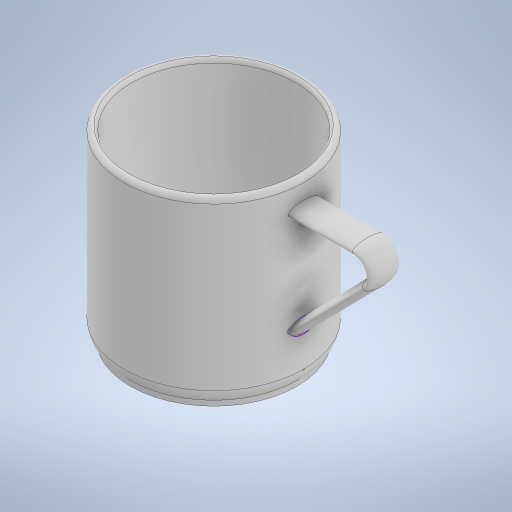
# Autodesk Inventor part: Lab No. 2
Saved by Autodesk Inventor 2024 (Build 280153000, 153)
## iProperties
Created: 2024-02-22
Part Number: Lab No. 2
Material: Generic
Document SubType Name: Modeling
Designer: Admin
Density: 1 g/cm^3
Appearance: Default
Author: Admin
Autodesk Inventor part; units mm, degrees
sketch "Sketch1" plane through (0, 0, 0) normal (0, 0, 1) x (1, 0, 0)
  line L0 (0, 0) -> (0, 70)
  line L1 (0, 70) -> (-35, 70)
  line L2 (-35, 70) -> (-35, 5)
  line L3 (0, 0) -> (-32.5, 0)
  arc A0 (-35, 5) -> (-32.5, 0) centre (-28.75, 5) ccw
  dimension "d0" = 70
  dimension "d1" = 35
  dimension "d2" = 65
  dimension "d3" = 32.5
  constraints: 8 end point, 2 perpendicular, 2 point on circle, 1 centre point, 1 horizontal, 1 tangent, 1 vertical
  measures "d0" distance of L0.start L0.end
  measures "d1" distance of L0.end L1.end
  measures "d2" distance of L1.end L2.end
  measures "d3" distance of L0.start L3.end
revolve "Revolution1" add sketch "Sketch1" angle 360 about axis through (0, 0, 0) along (0, 1, 0)
shell "Shell1" thickness 3 removed faces 1 at (-0.2748, 70, -9.3581)
sketch "Sketch2" plane through (0, 0, 0) normal (0, 0, 1) x (1, 0, 0)
  line L0 (35, 60) -> (60, 60)
  line L1 (35, 20) -> (64.0906, 49.6106)
  line L2 (35, 5) -> (35, 70) projected
  arc A0 (64.0906, 49.6106) -> (60, 60) centre (60, 54) ccw
  constraints: 4 end point, 2 point on circle, 1 centre point
ref_plane "Work Plane1" through (35, 60, 0) normal (1, 0, 0) x (0, 1, 0)
sketch "Sketch3" plane through (35, 60, 0) normal (1, 0, 0) x (0, 1, 0)
  ellipse E0 centre (0, 0) end of major axis (0, -6) minor radius 2
  point P0 (-60, 0)
  constraints: 2 other
ref_plane "Work Plane2" through (35, 5, 0) normal (1, 0, 0) x (0, 1, 0)
sketch "Sketch4" plane through (35, 5, 0) normal (1, 0, 0) x (0, 1, 0)
  point P0 (-5, 0)
ref_plane "Work Plane3" through (35, 20, 0) normal (1, 0, 0) x (0, 1, 0)
sketch "Sketch5" plane through (35, 20, 0) normal (1, 0, 0) x (0, 1, 0)
  ellipse E0 centre (0, 0) end of major axis (0, -5) minor radius 3
  point P0 (-20, 0)
  constraints: 2 other
sweep "Sweep1" add profiles "Sketch3" path "Sketch2" path curves L0 A0 L1
fillet "Fillet1" radius 2 2 edges at (35, 70, 0) (32, 70, 0)
sketch "Sketch6" plane through (0, 0, 0) normal (0, -1, 0) x (1, 0, 0)
  circle A0 centre (0, 0) radius 31
  circle A1 centre (0, 0) radius 32.5
  dimension "d34" = 62
  dimension "d35" = 65
  constraints: 2 centre point, 2 coincident
  measures "d34" diameter of A0
  measures "d35" diameter of A1
extrude "Extrusion1" add sketch "Sketch6" along normal blind 2 contours A0 | A1
body "Solid1"
